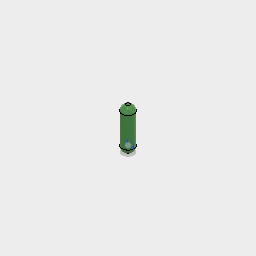
leg_Part_1 (Autodesk Fusion 360 design; units mm, degrees)
Autodesk Fusion 360 part; units mm, degrees
sketch "Sketch1" plane through (0, 0, 0) normal (0, 0, 1) x (1, 0, 0)
  line L0 (0, 0) -> (0, 4.8)
  line L1 (0, 0) -> (5, 0)
  line L2 (0, 4.8) -> (1.4, 4.8)
  arc A0 (5, 0) -> (1.4, 4.8) centre (0, 0) ccw
  dimension "d1" = 10
  dimension "d2" = 4.8
  dimension "d3" = 5
  measures "d1" diameter of A0
  measures "d2" distance of L0.start L0.end
  measures "d3" distance of L0.start L1.end
cylinder "CylinderPrimitive1" add diameter 10 height 25 placed x (1, 0, 0) y (0, 0, -1) z (0, 1, 0) at (0, 0, 0) makes body 1
revolve "Revolve1" add sketch "Sketch1" angle 360 about axis through (0, -25, 0) along (0, 1, 0) separate body makes body 2 in component "leg_1_Part_1_bottom"
sketch "sketch 1831" plane through (0, 0, 0) normal (0, 0, 1) x (1, 0, 0)
  line L0 (0, 0) -> (0, 4.8)
  line L1 (0, 0) -> (5, 0)
  arc A0 (5, 0) -> (1.4, 4.8) centre (0, 0) ccw
  line L2 (0, 4.8) -> (1.4, 4.8)
  line L3 (0, 0) -> (0, 4.8)
  line L4 (0, 0) -> (0, 4.8)
revolve "Revolve1'" add sketch "sketch 1831" angle 360 about axis through (0, 0, 0) along (0, -1, 0) separate body makes body 3 in component "leg_1_Part_1_top"
component "leg_1_Part_1_bottom" placed x (1, 0, 0) y (0, 1, 0) z (0, 0, 1) at (0, 25, 0)
component "leg_1_Part_1_top" placed x (1, 0, 0) y (0, -1, 0) z (0, 0, -1) at (0, 0, 0)
